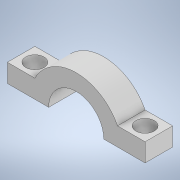
# Autodesk Inventor part: printHeadMount
Saved by Autodesk Inventor 2020 (Build 240168000, 168)
## iProperties
Created: 2020-02-03
Part Number: printHeadMount
Material: Generic
Document SubType Name: Modeling
Designer: PAB
Density: 1 g/cm^3
Appearance: Default
Author: PAB
Autodesk Inventor part; units mm, degrees
ref_plane "YZ Plane" through (0, 0, 0) normal (1, 0, 0) x (0, 1, 0)
ref_plane "XZ Plane" through (0, 0, 0) normal (0, 1, 0) x (-1, 0, 0)
ref_plane "XY Plane" through (0, 0, 0) normal (0, 0, 1) x (1, 0, 0)
sketch "Sketch1" plane through (0, 0, 0) normal (0, 1, 0) x (-1, 0, 0)
  line L0 (15, 6) -> (-15, 6)
  line L1 (-15, 6) -> (-15, 0)
  line L2 (-15, 0) -> (15, 0)
  line L3 (15, 0) -> (15, 6)
  point P0 (0, 0)
  dimension "d0" = 30
  constraints: 8 end point, 2 parallel, 1 horizontal, 1 perpendicular
  measures "d0" distance of L2.end L1.end
extrude "Extrusion1" add sketch "Sketch1" along normal blind 10
sketch "Sketch2" plane through (-15, 0, 6) normal (0, 0, 1) x (1, 0, 0)
  circle A0 centre (15, 0) radius 6
  line L0 (30, 10) -> (0, 10) projected
  line L1 (30, 10) -> (24, 10)
  line L2 (24, 10) -> (24, 4)
  line L3 (24, 4) -> (30, 4)
  line L4 (30, 4) -> (30, 10)
  line L5 (0, 0) -> (0, 10) projected
  line L6 (0, 10) -> (6, 10)
  line L7 (6, 10) -> (6, 4)
  line L8 (6, 4) -> (0, 4)
  line L9 (0, 4) -> (0, 10)
  arc A1 (24, 4) -> (6, 4) centre (15, -0.5678) ccw
  line L10 (6, 10) -> (24, 10)
  dimension "d3" = 12
  dimension "d4" = 6
  dimension "d5" = 6
  dimension "d6" = 6
  constraints: 18 end point, 4 parallel, 3 horizontal, 2 centre point, 2 perpendicular, 2 point on circle, 1 coincident
  measures "d3" diameter of A0
  measures "d4" distance of L3.end L2.end
  measures "d5" distance of L2.end L1.end
  measures "d6" distance of L7.end L8.end
extrude "Extrusion2" cut sketch "Sketch2" against normal blind 10
sketch "Sketch3" plane through (0, 0, 0) normal (0, -1, 0) x (1, 0, 0)
  circle A0 centre (-12, 3) radius 2
  circle A1 centre (12, 3) radius 2
  point P0 (0, 0)
  dimension "d9" = 4
  dimension "d10" = 4
  constraints: 2 centre point
  measures "d9" diameter of A0
  measures "d10" diameter of A1
extrude "Extrusion3" cut sketch "Sketch3" against normal blind 10
body "Solid1"
